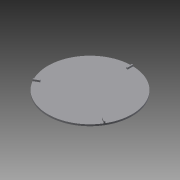
# Autodesk Inventor part: deltabot base
Saved by Autodesk Inventor 2015 SP2 (Build 190223200, 223)
## iProperties
Created: 2015-05-24
Part Number: deltabot base
Material: Generic
Document SubType Name: Modeling
Designer: caleb
Density: 1 g/cm^3
Appearance: Default
Author: caleb
Autodesk Inventor part; units mm, degrees
ref_plane "YZ Plane" through (0, 0, 0) normal (1, 0, 0) x (0, 1, 0)
ref_plane "XZ Plane" through (0, 0, 0) normal (0, 1, 0) x (-1, 0, 0)
ref_plane "XY Plane" through (0, 0, 0) normal (0, 0, 1) x (1, 0, 0)
sketch "Sketch1" plane through (0, 0, 0) normal (0, 0, 1) x (1, 0, 0)
  circle A0 centre (0, 0) radius 76.2
  dimension "d0" = 152.4
  constraints: 1 centre point, 1 coincident
  measures "d0" diameter of A0
extrude "Extrusion1" add sketch "Sketch1" along normal blind 3
sketch "Sketch2" plane through (0, 0, 3) normal (0, 0, 1) x (1, 0, 0)
  circle A0 centre (0, 0) radius 76.2 construction
  circle A1 centre (0, 0) radius 76.2 construction
  line L0 (2, 76.1737) -> (2, 66.1737)
  line L1 (2, 66.1737) -> (0, 66.1737)
  line L2 (0, 66.1737) -> (0, 76.2)
  arc A2 (2, 76.1737) -> (0, 76.2) centre (0, 0) ccw
  dimension "d5" = 2
  dimension "d6" = 10
  constraints: 6 end point, 2 perpendicular, 2 point on circle, 1 centre point, 1 coincident, 1 concentric, 1 point on line, 1 vertical
  measures "d5" distance of L0.end L1.end
  measures "d6" distance of L0.start L0.end
extrude "Extrusion2" add sketch "Sketch2" along normal blind 3
pattern_circular "Circular Pattern1" count 3 over 360 about axis through (0, 0, -10) along (0, 0, 1) of "Extrusion2"
body "Solid1"
